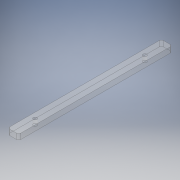
# Autodesk Inventor part: ToslinkHalter
Saved by Autodesk Inventor 2019 (Build 230136000, 136)
## iProperties
Created: 2018-05-15
Part Number: ToslinkHalter
Material: Polycarbonate, Clear
Document SubType Name: Modeling
Designer: Phil Erle
Density: 1.2 g/cm^3
Appearance: Polycarbonate - Clear
Author: Phil Erle
Autodesk Inventor part; units mm, degrees
ref_plane "YZ Plane" through (0, 0, 0) normal (1, 0, 0) x (0, 1, 0)
ref_plane "XZ Plane" through (0, 0, 0) normal (0, 1, 0) x (-1, 0, 0)
ref_plane "XY Plane" through (0, 0, 0) normal (0, 0, 1) x (1, 0, 0)
sketch "Sketch1" plane through (0, 0, 0) normal (0, 0, 1) x (1, 0, 0)
  line L0 (-5, -70) -> (5, -70)
  line L1 (5, -70) -> (5, 70)
  line L2 (5, 70) -> (-5, 70)
  line L3 (-5, 70) -> (-5, -70)
  line L4 (-5, -70) -> (5, 70) construction
  line L5 (5, -70) -> (-5, 70) construction
  point P0 (0, 0)
  dimension "d0" = 10
  dimension "d1" = 140
  constraints: 12 end point, 2 midpoint, 2 parallel, 1 horizontal, 1 perpendicular
  measures "d0" distance of L2.end L1.end
  measures "d1" distance of L1.end L0.end
extrude "Extrusion1" add sketch "Sketch1" along normal blind 5
sketch "Sketch2" plane through (0, 0, 5) normal (0, 0, 1) x (1, 0, 0)
  line L0 (0, 50) -> (0, -50) construction
  point P0 (0, 0)
  point P1 (0, 0)
  dimension "d4" = 100
  constraints: 3 coincident, 2 end point, 1 midpoint, 1 vertical, 1 vertical alignment
  measures "d4" distance of L0.start L0.end
hole "Hole1" at (0, 50, 5) at (0, -50, 5) direction (0, 0, -1) diameter 3.4 depth 8 tip angle 118 clearance for "Countersunk Flat Head Screw DIN EN ISO 2009" size "M3" standard "DIN"
fillet "Fillet1" radius 2 4 edges at (5, 70, 2.5) (-5, 70, 2.5) (5, -70, 2.5) (-5, -70, 2.5)
body "Solid1"
